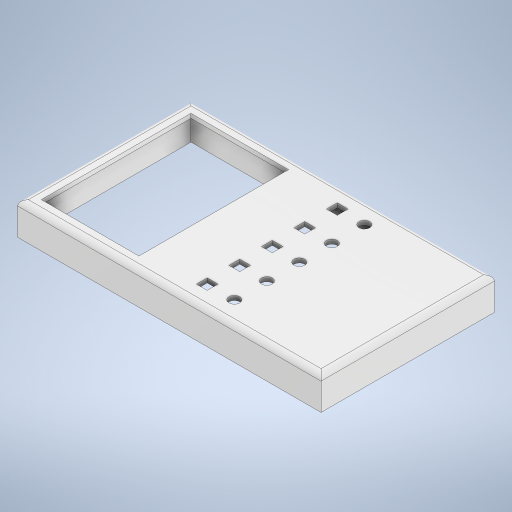
# Autodesk Inventor part: CaseTop
Saved by Autodesk Inventor 2023 (Build 270158000, 158)
## iProperties
Created: 2022-11-17
Part Number: CaseTop
Material: PC/ABS Plastic
Document SubType Name: Modeling
Designer: spfow
Density: 0.357273 g/cm^3
Appearance: Smooth - White
Author: spfow
Autodesk Inventor part; units mm, degrees
ref_plane "YZ Plane" through (0, 0, 0) normal (1, 0, 0) x (0, 1, 0)
ref_plane "XZ Plane" through (0, 0, 0) normal (0, 1, 0) x (-1, 0, 0)
ref_plane "XY Plane" through (0, 0, 0) normal (0, 0, 1) x (1, 0, 0)
sketch "Sketch1" plane through (0, 0, 0) normal (0, 1, 0) x (-1, 0, 0)
  line L0 (0, 0) -> (177.8, 0)
  line L1 (177.8, 0) -> (177.8, -101.6)
  line L2 (177.8, -101.6) -> (0, -101.6)
  line L3 (0, -101.6) -> (0, 0)
  point P0 (177.8, -50.8)
  point P1 (88.9, 0)
  point P2 (0, -50.8)
  dimension "d0" = 177.8
  dimension "d1" = 101.6
  constraints: 8 end point, 3 midpoint, 2 parallel, 1 horizontal, 1 perpendicular
  measures "d0" distance of L1.end L2.end
  measures "d1" distance of L0.end L1.end
extrude "Extrusion1" add sketch "Sketch1" along normal blind 19.05
fillet "Fillet1" radius 3.175 4 edges at (-88.9, 19.05, 0) (-177.8, 19.05, -50.8) (-88.9, 19.05, -101.6) (0, 19.05, -50.8)
sketch "Sketch2" plane through (0, 19.05, 0) normal (0, 1, 0) x (1, 0, 0)
  line L0 (-170.815, 6.985) -> (-113.665, 6.985)
  line L1 (-113.665, 6.985) -> (-113.665, 94.615)
  line L2 (-113.665, 94.615) -> (-170.815, 94.615)
  line L3 (-170.815, 94.615) -> (-170.815, 6.985)
  line L4 (-177.8, 0) -> (0, 0) projected
  line L5 (-177.8, 101.6) -> (-177.8, 0) projected
  line L6 (-82.55, 9.525) -> (-76.2, 9.525)
  line L7 (-76.2, 9.525) -> (-76.2, 15.875)
  line L8 (-76.2, 15.875) -> (-82.55, 15.875)
  line L9 (-82.55, 15.875) -> (-82.55, 9.525)
  line L10 (0, 0) -> (0, 101.6) projected
  line L11 (-82.55, 28.575) -> (-76.2, 28.575)
  line L12 (-76.2, 28.575) -> (-76.2, 34.925)
  line L13 (-76.2, 34.925) -> (-82.55, 34.925)
  line L14 (-82.55, 34.925) -> (-82.55, 28.575)
  line L15 (-82.55, 47.625) -> (-76.2, 47.625)
  line L16 (-76.2, 47.625) -> (-76.2, 53.975)
  line L17 (-76.2, 53.975) -> (-82.55, 53.975)
  line L18 (-82.55, 53.975) -> (-82.55, 47.625)
  line L19 (-82.55, 66.675) -> (-76.2, 66.675)
  line L20 (-76.2, 66.675) -> (-76.2, 73.025)
  line L21 (-76.2, 73.025) -> (-82.55, 73.025)
  line L22 (-82.55, 73.025) -> (-82.55, 66.675)
  line L23 (-82.55, 85.725) -> (-76.2, 85.725)
  line L24 (-76.2, 85.725) -> (-76.2, 92.075)
  line L25 (-76.2, 92.075) -> (-82.55, 92.075)
  line L26 (-82.55, 92.075) -> (-82.55, 85.725)
  circle A0 centre (-63.5, 12.7) radius 3.175
  circle A1 centre (-63.5, 31.75) radius 3.175
  circle A2 centre (-63.5, 50.8) radius 3.175
  circle A3 centre (-63.5, 69.85) radius 3.175
  circle A4 centre (-63.5, 88.9) radius 3.175
  line L27 (0, 101.6) -> (-177.8, 101.6) projected
  point P0 (-79.375, 15.875)
  point P1 (-79.375, 28.575)
  point P2 (-79.375, 34.925)
  point P3 (-79.375, 47.625)
  dimension "d47" = 87.63
  dimension "d48" = 57.15
  dimension "d49" = 6.985
  dimension "d50" = 6.985
  dimension "d51" = 6.35
  dimension "d52" = 6.35
  dimension "d53" = 9.525
  dimension "d54" = 76.2
  dimension "d55" = 6.35
  dimension "d56" = 6.35
  dimension "d57" = 6.35
  dimension "d58" = 6.35
  dimension "d59" = 6.35
  dimension "d60" = 6.35
  dimension "d61" = 6.35
  dimension "d62" = 6.35
  dimension "d63" = 12.7
  dimension "d64" = 12.7
  dimension "d65" = 12.7
  dimension "d66" = 12.7
  dimension "d67" = 76.2
  dimension "d68" = 6.35
  dimension "d69" = 6.35
  dimension "d70" = 6.35
  dimension "d71" = 6.35
  dimension "d72" = 6.35
  dimension "d73" = 63.5
  dimension "d74" = 63.5
  dimension "d75" = 63.5
  dimension "d76" = 63.5
  dimension "d77" = 63.5
  dimension "d78" = 12.7
  dimension "d79" = 19.05
  dimension "d80" = 19.05
  dimension "d81" = 19.05
  dimension "d82" = 19.05
  constraints: 48 end point, 12 parallel, 6 horizontal, 6 perpendicular, 6 point on line, 5 centre point, 4 midpoint
  measures "d47" distance of L2.end L0.start
  measures "d48" distance of L0.start L0.end
  measures "d49" distance between parallel lines of L4 L0
  measures "d50" distance between parallel lines of L5 L3
  measures "d51" distance of L8.end L7.end
  measures "d52" distance of L6.end L7.end
  measures "d53" distance between parallel lines of L4 L6
  measures "d54" distance between parallel lines of L10 L7
  measures "d55" distance of L12.end L13.end
  measures "d56" distance of L16.end L17.end
  measures "d57" distance of L20.end L21.end
  measures "d58" distance of L24.end L25.end
  measures "d59" distance of L13.end L11.start
  measures "d60" distance of L15.start L17.end
  measures "d61" distance of L21.end L19.start
  measures "d62" distance of L25.end L23.start
  measures "d63" distance of point (-79.375, 15.875) point (-79.375, 28.575)
  measures "d64" distance of point (-79.375, 34.925) point (-79.375, 47.625)
  measures "d65" distance between parallel lines of L17 L19
  measures "d66" distance between parallel lines of L21 L23
  measures "d67" distance from line of L10 L12.end
  measures "d68" diameter of A0
  measures "d69" diameter of A1
  measures "d70" diameter of A2
  measures "d71" diameter of A3
  measures "d72" diameter of A4
  measures "d73" distance from line of L10 A0.centre
  measures "d74" distance from line of L10 A1.centre
  measures "d75" distance from line of L10 A2.centre
  measures "d76" distance from line of L10 A3.centre
  measures "d77" distance from line of L10 A4.centre
  measures "d78" distance from line of L27 A4.centre
  measures "d79" distance of A3.centre A4.centre
  measures "d80" distance of A3.centre A2.centre
  measures "d81" distance of A2.centre A1.centre
  measures "d82" distance of A1.centre A0.centre
shell "Shell2" thickness 2.54 removed faces 1 at (-59.2667, 0, -33.8667)
extrude "Extrusion2" cut sketch "Sketch2" against normal blind 19.05 contours L3 L2 L1 L0 | L9 L8 L7 L6 | L14 L13 L12 L11 | L18 L17 L16 L15 | L22 L21 L20 L19 | L26 L25 L24 L23 | A0 | A1 | A2 | A3 | A4
body "Solid1"
